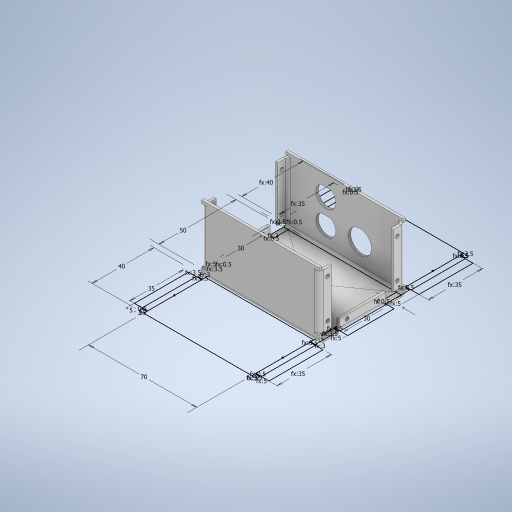
# Autodesk Inventor part: Bottom
Saved by Autodesk Inventor 2024 (Build 280153000, 153)
## iProperties
Created: 2025-10-28
Part Number: Bottom
Material: 일반
Document SubType Name: Sheet Metal
Designer: alexi
Density: 1 g/cm^3
Sheet Metal Rule: 기본값_mm
Appearance: 기본값
Flat Pattern Width: 8.7 cm
Flat Pattern Length: 13.7 cm
Flat Pattern Area: 119.19 cm^2
Sheet Metal Width: 87.000 mm
Sheet Metal Length: 137.000 mm
Sheet Metal Area: 11919.000 mm^2
Author: alexi
Autodesk Inventor part; units mm, degrees
ref_plane "YZ Plane" through (0, 0, 0) normal (1, 0, 0) x (0, 1, 0)
ref_plane "XZ Plane" through (0, 0, 0) normal (0, 1, 0) x (-1, 0, 0)
ref_plane "XY Plane" through (0, 0, 0) normal (0, 0, 1) x (1, 0, 0)
sketch "Holes" plane through (0, 0, 0) normal (0, 0, 1) x (1, 0, 0)
  circle A0 centre (-13.7245, -10.9519) radius 4.4501 construction
  circle A1 centre (-13.7245, -26.9514) radius 4.0754 construction
  circle A2 centre (-35.7245, -25.0992) radius 0.9 construction
  point P0 (-21.0578, -21.0008)
sketch "PCB Holes" plane through (0, 0, 0) normal (0, 0, 1) x (1, 0, 0)
  circle A0 centre (-19.0196, -39.1634) radius 8.8876 construction
  circle A1 centre (2.9804, -41.0157) radius 7.94 construction
  circle A2 centre (2.9804, -25.0162) radius 7.94 construction
  line L0 (20.9804, -49.4134) -> (-39.0196, -49.4134) construction
  line L1 (20.9804, -50.0372) -> (-39.0196, -50.0372) construction
  line L2 (-39.0196, -50.0372) -> (-39.0196, -49.4134) construction
  line L3 (20.9804, -50.0372) -> (20.9804, -49.4134) construction
  arc A3 (-0.2367, -19.4662) -> (6.1975, -19.4662) centre (2.9804, -25.0162) ccw
  line L4 (-0.2367, -19.4662) -> (6.1975, -19.4662)
  arc A4 (-0.2367, -35.4657) -> (6.1975, -35.4657) centre (2.9804, -41.0157) ccw
  line L5 (-0.2367, -35.4657) -> (6.1975, -35.4657)
  circle A5 centre (-19.0196, -39.1634) radius 7.5
  point P0 (-3.4949, -37.3055)
  dimension "d205" = 6.415
  dimension "d206" = 5.55
  dimension "d207" = 6.415
  dimension "d208" = 5.55
  dimension "d209" = 15
  measures "d205" radius of A3
  measures "d206" distance from line of A2.centre L4
  measures "d207" radius of A4
  measures "d208" distance from line of A1.centre L5
  measures "d209" diameter of A5
sketch "스케치1" plane through (0, 0, 0) normal (0, 1, 0) x (-1, 0, 0)
  line L0 (35, -25) -> (-35, -25)
  line L1 (-35, -25) -> (-35, 25)
  line L2 (-35, 25) -> (35, 25)
  line L3 (35, 25) -> (35, -25)
  line L4 (35, -25) -> (-35, -25)
  line L5 (-35, -25) -> (-35, -28.5)
  line L6 (-35, -28.5) -> (35, -28.5)
  line L7 (35, -28.5) -> (35, -25)
  line L8 (35, 25) -> (-35, 25)
  line L9 (-35, 25) -> (-35, 28.5)
  line L10 (-35, 28.5) -> (35, 28.5)
  line L11 (35, 28.5) -> (35, 25)
  line L12 (35, 28.5) -> (-35, 28.5)
  line L13 (-35, 28.5) -> (-35, 68.5)
  line L14 (-35, 68.5) -> (35, 68.5)
  line L15 (35, 68.5) -> (35, 28.5)
  line L16 (35, -28.5) -> (-35, -28.5)
  line L17 (-35, -28.5) -> (-35, -68.5)
  line L18 (-35, -68.5) -> (35, -68.5)
  line L19 (35, -68.5) -> (35, -28.5)
  line L20 (35, 25) -> (-35, -25) construction
  line L21 (35, -25) -> (-35, 25) construction
  line L22 (35, 26.75) -> (-35, 26.75) construction
  line L23 (35, -26.75) -> (-35, -26.75) construction
  line L24 (35, -15) -> (38.5, -15)
  line L25 (38.5, -15) -> (38.5, 15)
  line L26 (38.5, 15) -> (35, 15)
  line L27 (35, 15) -> (35, -15)
  line L28 (-35, -15) -> (-38.5, -15)
  line L29 (-38.5, -15) -> (-38.5, 15)
  line L30 (-38.5, 15) -> (-35, 15)
  line L31 (-35, 15) -> (-35, -15)
  line L32 (38.5, -15) -> (43.5, -15)
  line L33 (43.5, -15) -> (43.5, 15)
  line L34 (43.5, 15) -> (38.5, 15)
  line L35 (38.5, 15) -> (38.5, -15)
  line L36 (-38.5, -15) -> (-43.5, -15)
  line L37 (-43.5, -15) -> (-43.5, 15)
  line L38 (-43.5, 15) -> (-38.5, 15)
  line L39 (-38.5, 15) -> (-38.5, -15)
  line L40 (35, -66) -> (38.5, -66)
  line L41 (38.5, -66) -> (38.5, -31)
  line L42 (38.5, -31) -> (35, -31)
  line L43 (35, -31) -> (35, -66)
  line L44 (-35, -66) -> (-38.5, -66)
  line L45 (-38.5, -66) -> (-38.5, -31)
  line L46 (-38.5, -31) -> (-35, -31)
  line L47 (-35, -31) -> (-35, -66)
  line L48 (35, 31) -> (38.5, 31)
  line L49 (38.5, 31) -> (38.5, 66)
  line L50 (38.5, 66) -> (35, 66)
  line L51 (35, 66) -> (35, 31)
  line L52 (38.5, 31) -> (43.5, 31)
  line L53 (43.5, 31) -> (43.5, 66)
  line L54 (43.5, 66) -> (38.5, 66)
  line L55 (38.5, 66) -> (38.5, 31)
  line L56 (-38.5, -66) -> (-43.5, -66)
  line L57 (-43.5, -66) -> (-43.5, -31)
  line L58 (-43.5, -31) -> (-38.5, -31)
  line L59 (-38.5, -31) -> (-38.5, -66)
  line L60 (38.5, -66) -> (43.5, -66)
  line L61 (43.5, -66) -> (43.5, -31)
  line L62 (43.5, -31) -> (38.5, -31)
  line L63 (38.5, -31) -> (38.5, -66)
  line L64 (-35, 31) -> (-38.5, 31)
  line L65 (-38.5, 31) -> (-38.5, 66)
  line L66 (-38.5, 66) -> (-35, 66)
  line L67 (-35, 66) -> (-35, 31)
  line L68 (-38.5, 31) -> (-43.5, 31)
  line L69 (-43.5, 31) -> (-43.5, 66)
  line L70 (-43.5, 66) -> (-38.5, 66)
  line L71 (-38.5, 66) -> (-38.5, 31)
  line L72 (-38, 30.5) -> (-38, 15.5)
  line L73 (-38, 15.5) -> (-35, 15.5)
  line L74 (-35, 15.5) -> (-35, 25)
  line L75 (-38, -15.5) -> (-35, -15.5)
  line L76 (38, -15.5) -> (35, -15.5)
  line L77 (38, 30.5) -> (38, 15.5)
  line L78 (38, 15.5) -> (35, 15.5)
  line L79 (35, 15.5) -> (35, 25)
  line L80 (-38, 30.5) -> (-35, 30.5)
  line L81 (-35, 68.5) -> (-38, 68.5)
  line L82 (-38, 68.5) -> (-38, 66.5)
  line L83 (-38, 66.5) -> (-35, 66.5)
  line L84 (-35, 66.5) -> (-35, 68.5)
  line L85 (35, 68.5) -> (38, 68.5)
  line L86 (38, 68.5) -> (38, 66.5)
  line L87 (38, 66.5) -> (35, 66.5)
  line L88 (35, 66.5) -> (35, 68.5)
  line L89 (38, 30.5) -> (35, 30.5)
  line L90 (-38, -15.5) -> (-38, -30.5)
  line L91 (-38, -30.5) -> (-35, -30.5)
  line L92 (-35, -68.5) -> (-38, -68.5)
  line L93 (-38, -68.5) -> (-38, -66.5)
  line L94 (-38, -66.5) -> (-35, -66.5)
  line L95 (-35, -66.5) -> (-35, -68.5)
  line L96 (35, -68.5) -> (38, -68.5)
  line L97 (38, -68.5) -> (38, -66.5)
  line L98 (38, -66.5) -> (35, -66.5)
  line L99 (35, -66.5) -> (35, -68.5)
  line L100 (38, -15.5) -> (38, -30.5)
  line L101 (38, -30.5) -> (35, -30.5)
  line L102 (-38, 25) -> (38, 25)
  line L103 (-38, -25) -> (38, -25)
  point P0 (0, 0)
  point P1 (0, 0)
  point P2 (35, 0)
  point P3 (-35, 0)
  point P4 (-35, 15)
  point P5 (35, 15)
  point P6 (35, -48.5)
  point P7 (-35, -48.5)
  point P8 (35, 48.5)
  point P9 (-35, 48.5)
  point P10 (-35, -31)
  point P11 (-35, 66)
  point P12 (35, 66)
  point P13 (-35, 15.5)
  point P14 (35, 15.5)
  dimension "d0" = 50
  dimension "d1" = 70
  dimension "d2" = 3.5
  dimension "d3" = 3.5
  dimension "d4" = 40
  dimension "d5" = 40
  dimension "d19" = 30
  dimension "d20" = 30
  dimension "d21" = 3.5
  dimension "d22" = 3.5
  dimension "d23" = 5
  dimension "d24" = 5
  dimension "d37" = 3.5
  dimension "d38" = 3.5
  dimension "d40" = 3.5
  dimension "d41" = 5
  dimension "d43" = 5
  dimension "d44" = 5
  dimension "d45" = 3.5
  dimension "d46" = 5
  dimension "d47" = 35
  dimension "d48" = 35
  dimension "d49" = 35
  dimension "d50" = 35
  dimension "d169" = 0.5
  dimension "d170" = 3
  dimension "d171" = 0.5
  dimension "d172" = 0.5
  dimension "d173" = 0.5
  dimension "d174" = 0.5
  dimension "d175" = 0.5
  dimension "d176" = 0.5
  dimension "d177" = 0.5
  dimension "d178" = 0.5
  dimension "d179" = 0.5
  dimension "d180" = 0.5
  dimension "d181" = 0.5
  dimension "d182" = 3
  dimension "d185" = 3
  dimension "d189" = 3
  dimension "d196" = 3
  dimension "d197" = 3
  constraints: 208 end point, 44 parallel, 23 horizontal, 22 perpendicular, 19 point on line, 18 midpoint, 3 vertical, 1 coincident
  measures "d0" distance of L2.end L0.start
  measures "d1" distance of L13.end L14.end
  measures "d2" distance of L10.end L2.end
  measures "d3" distance of L6.end L0.start
  measures "d4" distance of L14.end L10.end
  measures "d5" distance of L18.end L6.end
  measures "d19" distance of L24.end L25.end
  measures "d20" distance of L28.end L29.end
  measures "d21" distance of L25.end L26.end
  measures "d22" distance of L29.end L30.end
  measures "d23" distance of L25.end L33.end
  measures "d24" distance of L29.end L37.end
  measures "d37" distance of L40.start L40.end
  measures "d38" distance of L44.start L44.end
  measures "d40" distance of L49.end L50.end
  measures "d41" distance of L49.end L53.end
  measures "d43" distance of L41.end L61.end
  measures "d44" distance of L45.end L57.end
  measures "d45" distance of L65.end L66.end
  measures "d46" distance of L69.end L65.end
  measures "d47" distance of L52.end L53.end
  measures "d48" distance of L68.end L69.end
  measures "d49" distance of L60.end L61.end
  measures "d50" distance of L56.end L57.end
  measures "d169" distance between parallel lines of L50 L87
  measures "d170" distance of L14.end L85.end
  measures "d171" distance between parallel lines of L66 L83
  measures "d172" distance between parallel lines of L64 L80
  measures "d173" distance between parallel lines of L48 L89
  measures "d174" distance between parallel lines of L26 L78
  measures "d175" distance between parallel lines of L30 L73
  measures "d176" distance between parallel lines of L28 L75
  measures "d177" distance between parallel lines of L91 L46
  measures "d178" distance between parallel lines of L44 L94
  measures "d179" distance between parallel lines of L40 L98
  measures "d180" distance between parallel lines of L24 L76
  measures "d181" distance between parallel lines of L42 L101
  measures "d182" distance of L13.end L81.end
  measures "d185" distance of L18.end L96.end
  measures "d189" distance of L72.start L80.end
  measures "d196" distance between parallel lines of L100 L3
  measures "d197" distance between parallel lines of L77 L11
extrude "판1" add sketch "스케치1" against normal blind 1.5
fold "접기11" angle 90 bend radius 1.5 thickness 1.5 k factor 0.44 line from (38.5, 0, 31) to (38.5, 0, 66) line at bend end moving side (1, 0, 0) folds toward (0, 1, 0)
fold "접기12" angle 90 bend radius 1.5 thickness 1.5 k factor 0.44 line from (-38.5, 0, 31) to (-38.5, 0, 66) line at bend end moving side (-1, 0, 0) folds toward (0, 1, 0)
fold "접기13" angle 90 bend radius 1.5 thickness 1.5 k factor 0.44 line from (38.5, 0, -15) to (38.5, 0, 15) line at bend end moving side (1, 0, 0) folds toward (0, 1, 0)
fold "접기14" angle 90 bend radius 1.5 thickness 1.5 k factor 0.44 line from (-38.5, 0, -15) to (-38.5, 0, 15) line at bend end moving side (-1, 0, 0) folds toward (0, 1, 0)
fold "접기15" angle 90 bend radius 1.5 thickness 1.5 k factor 0.44 line from (38.5, 0, -31) to (38.5, 0, -66) line at bend end moving side (1, 0, 0) folds toward (0, 1, 0)
fold "접기16" angle 90 bend radius 1.5 thickness 1.5 k factor 0.44 line from (-38.5, 0, -66) to (-38.5, 0, -31) line at bend end moving side (-1, 0, 0) folds toward (0, 1, 0)
fold "접기19" angle 90 bend radius 1.5 thickness 1.5 k factor 0.44 line from (38, 0, 25) to (-38, 0, 25) line at bend start moving side (0, 0, 1) folds toward (0, 1, 0)
fold "접기20" angle 90 bend radius 1.5 thickness 1.5 k factor 0.44 line from (38, 0, -25) to (-38, 0, -25) line at bend start moving side (0, 0, -1) folds toward (0, 1, 0)
sketch "스케치7" plane through (38, 41.6071, -28) normal (0, 0, -1) x (-1, 0, 0)
  line L0 (0, -41.6071) -> (76, -41.6071) projected
  line L1 (38, -41.6071) -> (38, -37.6071) construction
  circle A0 centre (28, -26.7334) radius 8.8876 construction
  circle A1 centre (50, -28.5856) radius 7.94 construction
  circle A2 centre (50, -12.5861) radius 7.94 construction
  line L2 (68, -36.9834) -> (8, -36.9834) construction
  line L3 (68, -37.6071) -> (8, -37.6071) construction
  line L4 (8, -37.6071) -> (8, -36.9834) construction
  line L5 (68, -37.6071) -> (68, -36.9834) construction
  arc A3 (46.7829, -7.0361) -> (53.2171, -7.0361) centre (50, -12.5861) ccw
  line L6 (46.7829, -7.0361) -> (53.2171, -7.0361)
  arc A4 (46.7829, -23.0356) -> (53.2171, -23.0356) centre (50, -28.5856) ccw
  line L7 (46.7829, -23.0356) -> (53.2171, -23.0356)
  circle A5 centre (28, -26.7334) radius 7.5
  dimension "d204" = 4
  constraints: 2 end point, 1 perpendicular, 1 other
extrude "돌출2" cut sketch "스케치7" against normal blind 10
sketch "스케치8" plane through (38.1071, 4.1071, 20) normal (1, 0, 0) x (0, 0, -1)
  line L0 (0, 35) -> (-5, 35) projected
  line L1 (-2.5, 35) -> (-2.5, 0) construction
  line L2 (-5, 0) -> (0, 0) projected
  line L3 (5, 2.3929) -> (5, -2.6071) projected
  line L4 (5, -0.1071) -> (35, -0.1071) construction
  line L5 (35, -2.6071) -> (35, 2.3929) projected
  line L6 (40, 0) -> (45, 0) projected
  line L7 (42.5, 0) -> (42.5, 35) construction
  line L8 (45, 35) -> (40, 35) projected
  point P0 (20, -4.1071)
  point P1 (-2.5, 30)
  point P2 (-2.5, 5)
  point P3 (10, -0.1071)
  point P4 (30, -0.1071)
  point P5 (42.5, 5)
  point P6 (42.5, 30)
  dimension "d212" = 5
  dimension "d213" = 5
  dimension "d214" = 5
  dimension "d215" = 5
  dimension "d216" = 5
  dimension "d217" = 5
  constraints: 6 end point, 6 midpoint, 6 point on line
  measures "d212" distance from line of L0 point (-2.5, 30)
  measures "d213" distance from line of L2 point (-2.5, 5)
  measures "d214" distance from line of L3 point (10, -0.107)
  measures "d215" distance from line of L5 point (30, -0.107)
  measures "d216" distance from line of L6 point (42.5, 5)
  measures "d217" distance from line of L8 point (42.5, 30)
hole "구멍3" at (38.1071, 34.1071, -22.5) at (38.1071, 34.1071, 22.5) at (38.1071, 9.1071, 22.5) at (38.1071, 4, 10) at (38.1071, 4, -10) at (38.1071, 9.1071, -22.5) direction (-1, 0, 0) diameter 2.459 depth 1.5 tip angle 118 thread size "M3x0.5" class "6H" standard "ANSI Metric M Profile"
sketch "스케치9" plane through (-38.1071, 4.1071, -20) normal (-1, 0, 0) x (0, 0, 1)
  line L0 (-5, 35) -> (0, 35) projected
  line L1 (-2.5, 35) -> (-2.5, 0) construction
  line L2 (-5, 0) -> (0, 0) projected
  line L3 (5, -2.6071) -> (5, 2.3929) projected
  line L4 (5, -0.1071) -> (35, -0.1071) construction
  line L5 (35, 2.3929) -> (35, -2.6071) projected
  line L6 (45, 0) -> (40, 0) projected
  line L7 (42.5, 0) -> (42.5, 35) construction
  line L8 (40, 35) -> (45, 35) projected
  point P0 (20, -4.1071)
  point P1 (-2.5, 30)
  point P2 (-2.5, 5)
  point P3 (10, -0.1071)
  point P4 (30, -0.1071)
  point P5 (42.5, 5)
  point P6 (42.5, 30)
  dimension "d225" = 5
  dimension "d226" = 5
  dimension "d227" = 5
  dimension "d228" = 5
  dimension "d229" = 5
  dimension "d230" = 5
  constraints: 6 end point, 6 midpoint, 6 point on line
  measures "d225" distance from line of L0 point (-2.5, 30)
  measures "d226" distance from line of L2 point (-2.5, 5)
  measures "d227" distance from line of L3 point (10, -0.107)
  measures "d228" distance from line of L5 point (30, -0.107)
  measures "d229" distance from line of L6 point (42.5, 5)
  measures "d230" distance from line of L8 point (42.5, 30)
hole "구멍4" at (-38.1071, 34.1071, -22.5) at (-38.1071, 9.1071, -22.5) at (-38.1071, 4, -10) at (-38.1071, 4, 10) at (-38.1071, 9.1071, 22.5) at (-38.1071, 34.1071, 22.5) direction (1, 0, 0) diameter 2.459 depth 1.5 tip angle 118 thread size "M3x0.5" class "6H" standard "ANSI Metric M Profile"
equation "\"d2\" = d40"
equation "\"d3\" = d40"
equation "\"d5\" = d4"
equation "\"d21\" = d40"
equation "\"d22\" = d40"
equation "\"d23\" = d41"
equation "\"d24\" = d41"
equation "\"d37\" = d40"
equation "\"d38\" = d40"
equation "\"d43\" = d41"
equation "\"d44\" = d41"
equation "\"d45\" = d40"
equation "\"d46\" = d41"
equation "\"d48\" = d47"
equation "\"d49\" = d47"
equation "\"d50\" = d47"
equation "\"d171\" = d169"
equation "\"d172\" = d169"
equation "\"d173\" = d169"
equation "\"d174\" = d169"
equation "\"d175\" = d169"
equation "\"d176\" = d169"
equation "\"d177\" = d169"
equation "\"d178\" = d169"
equation "\"d179\" = d169"
equation "\"d180\" = d169"
equation "\"d181\" = d169"
equation "\"d182\" = d170"
equation "\"d185\" = d170"
equation "\"d87\" = BendReliefWidth"
equation "\"d88\" = BendReliefDepth"
equation "\"d89\" = MinimumRemnant"
equation "\"d90\" = TransitionRadius"
equation "\"d93\" = BendReliefWidth"
equation "\"d94\" = BendReliefDepth"
equation "\"d95\" = MinimumRemnant"
equation "\"d96\" = TransitionRadius"
equation "\"d99\" = BendReliefWidth"
equation "\"d100\" = BendReliefDepth"
equation "\"d101\" = MinimumRemnant"
equation "\"d102\" = TransitionRadius"
equation "\"d105\" = BendReliefWidth"
equation "\"d106\" = BendReliefDepth"
equation "\"d107\" = MinimumRemnant"
equation "\"d108\" = TransitionRadius"
equation "\"d111\" = BendReliefWidth"
equation "\"d112\" = BendReliefDepth"
equation "\"d113\" = MinimumRemnant"
equation "\"d114\" = TransitionRadius"
equation "\"d117\" = BendReliefWidth"
equation "\"d118\" = BendReliefDepth"
equation "\"d119\" = MinimumRemnant"
equation "\"d120\" = TransitionRadius"
equation "\"TransitionRadius\" = BendRadius"
equation "\"BendReliefWidth\" = 1.5"
equation "\"BendReliefDepth\" = 0.75"
equation "\"MinimumRemnant\" = 3"
equation "\"BendRadius\" = 1.5"
